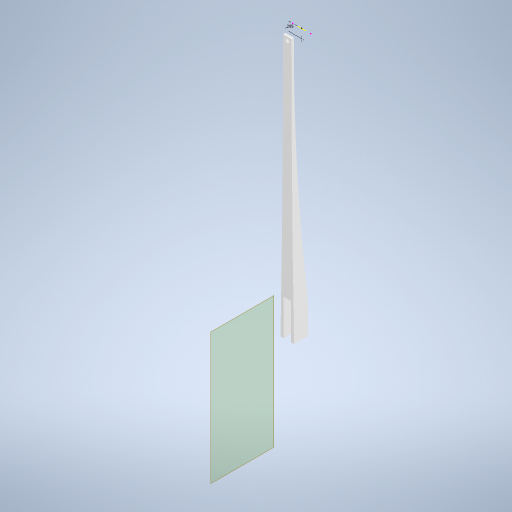
# Autodesk Inventor part: Halterung
Saved by Autodesk Inventor 2023 (Build 270158000, 158)
## iProperties
Created: 2023-02-18
Part Number: Halterung
Material: ABS Plastic
Document SubType Name: Modeling
Designer: phill
Density: 1.06 g/cm^3
Appearance: Smooth - White
Author: phill
Autodesk Inventor part; units mm, degrees
ref_plane "YZ Plane" through (0, 0, 0) normal (1, 0, 0) x (0, 1, 0)
ref_plane "XZ Plane" through (0, 0, 0) normal (0, 1, 0) x (-1, 0, 0)
sketch "Sketch2" plane through (0, 0, 0) normal (0, 0, 1) x (1, 0, 0)
  line L0 (0, 0) -> (0, -100) projected
  line L1 (0, 0) -> (6, 0) projected
  line L2 (6, -100) -> (6, 0) projected
  line L3 (0, -100) -> (6, -100) projected
  line L4 (10.5, -30) -> (-4.5, -30)
  line L5 (-4.5, -30) -> (-4.5, 190)
  line L6 (-4.5, 190) -> (10.5, 190)
  line L7 (10.5, 190) -> (10.5, -30)
  line L8 (6.5, 0.5) -> (-0.5, 0.5)
  line L9 (-0.5, 0.5) -> (-0.5, -100.5)
  line L10 (-0.5, -100.5) -> (6.5, -100.5)
  line L11 (6.5, -100.5) -> (6.5, 0.5)
  line L12 (6.5, 0.5) -> (-0.5, 0.5)
  line L13 (-0.5, 0.5) -> (-0.5, 190)
  line L14 (-0.5, 190) -> (6.5, 190)
  line L15 (6.5, 190) -> (6.5, 0.5)
  line L16 (0, -100) -> (0, 0) projected
  line L17 (0, 0) -> (6, 0) projected
  line L18 (6, 0) -> (6, -100) projected
  line L19 (-0.5, 175) -> (6.5, 175)
  line L20 (-4.5, 175) -> (-0.5, 175)
  line L21 (6.5, 175) -> (10.5, 175)
  circle A0 centre (3, -90) radius 1.5 projected
  arc A1 (-2.6174, -30) -> (-0.5, 190) centre (-11430.5, 190) ccw
  arc A2 (6.5, 190) -> (8.6174, -30) centre (11436.5, 190) ccw
  point P0 (3, -30)
  point P1 (3, 0)
  point P2 (3, 182.5)
  point P3 (3, 0)
  point P4 (3, 190)
  point P5 (3, 190)
  dimension "d0" = 30
  dimension "d1" = 15
  dimension "d2" = 220
  dimension "d3" = 0.5
  dimension "d8" = 7.5
  dimension "d10" = 22860
  dimension "d11" = 22860
  constraints: 30 end point, 5 horizontal, 5 midpoint, 4 parallel, 4 point on circle, 3 point on line, 2 centre point, 2 horizontal alignment, 2 perpendicular, 2 tangent, 2 vertical alignment, 1 coincident, 7 other
  measures "d0" distance between parallel lines of L1 L4
  measures "d1" distance between parallel lines of L5 L7
  measures "d2" distance between parallel lines of L6 L4
  measures "d3" distance between parallel lines of L11 L2
  measures "d8" distance from line of L6 point (3, 182.5)
  measures "d10" diameter of A1
  measures "d11" diameter of A2
extrude "Extrusion1" add sketch "Sketch2" against normal blind 4 contours L1 L2 L4 L0 | L0 L4 L9 L8 L11 L2 L1 | L4 A1 L20 L13 L9 | L11 L15 L21 A2 L4 | L13 L19 L15 L8 | A1 L13 L20 | L13 L6 L15 L19 | L21 L15 A2
sketch "Sketch3" plane through (0, 0, 0) normal (0, 0, 1) x (1, 0, 0)
  line L0 (10.5, -30) -> (10.5, 190) projected
  line L1 (6.5, 190) -> (6.5, 0.5) projected
  line L2 (6.5, -100.5) -> (6.5, 0.5) projected
  line L3 (-0.5, 0.5) -> (-0.5, -100.5) projected
  line L4 (-0.5, 0.5) -> (-0.5, 190) projected
  line L5 (6.5, 0.5) -> (-0.5, 0.5) projected
  line L6 (-4.5, -30) -> (10.5, -30) projected
  line L7 (-2.6174, -30) -> (8.6174, -30) projected
  line L8 (6.5, 190) -> (-0.5, 190) projected
  arc A0 (6.5, 190) -> (8.6174, -30) centre (11436.5, 190) ccw projected
  arc A1 (-2.6174, -30) -> (-0.5, 190) centre (-11430.5, 190) ccw projected
  point P0 (0, 0)
  point P1 (-0.5, -30)
  point P2 (6.5, -30)
  point P3 (-0.5, 190)
  point P4 (6.5, 190)
extrude "Extrusion2" add sketch "Sketch3" along normal blind 8
sketch "Sketch4" plane through (0, 0, -4) normal (0, 0, -1) x (-1, 0, 0)
  line L0 (0.5, 190) -> (-6.5, 190) projected
  point P0 (0, 0)
  point P1 (-3, 182.507)
  point P2 (4.5, 190)
  point P3 (-10.5, 190)
  point P4 (-3, 190)
  dimension "d9" = 7.493
  constraints: 1 midpoint, 1 vertical alignment
  measures "d9" distance from line of L0 point (-3, 182.507)
sketch "Sketch5" plane through (0, 0, -4) normal (0, 0, -1) x (-1, 0, 0)
  line L0 (-8.6174, -30) -> (2.6174, -30) projected
  line L1 (0.5, 190) -> (-6.5, 190) projected
  point P0 (0, 0)
  point P1 (-3, 187)
  point P2 (-3, -30)
  point P3 (-3, 190)
  dimension "d12" = 3
  constraints: 2 midpoint, 1 vertical alignment
  measures "d12" distance of point (-3, 190) point (-3, 187)
hole "Hole1" at (3, 187, -4) direction (0, 0, 1) diameter 3 end through all
ref_plane "Work Plane1" through (0, -50, 42.7167) normal (-1, 0, 0) x (0, 1, 0)
sketch "Sketch6" plane through (0, -50, 42.7167) normal (-1, 0, 0) x (0, 1, 0)
  arc A0 (20, 49.8247) -> (240, 36.7224) centre (235.5, 1814.7167) ccw
  line L0 (235.5, 46.7167) -> (238.5, 46.7167) projected
  line L1 (20, 46.7167) -> (240, 46.7167) projected
  line L2 (240, 46.7167) -> (20, 46.7167) projected
  line L3 (235.5, 34.7167) -> (235.5, 46.7167) projected
  line L4 (238.5, 34.7167) -> (238.5, 46.7167) projected
  line L5 (235.5, 34.7167) -> (235.5, 46.7167) projected
  line L6 (240, 46.7167) -> (240, 34.7167) projected
  line L7 (20, 46.7167) -> (240, 46.7167) projected
  line L8 (20, 34.7167) -> (20, 46.7167) projected
  line L9 (240, 34.7167) -> (20, 34.7167) projected
  point P0 (50, 42.7167)
  point P1 (47.1917, 46.7167)
  dimension "d20" = 2
  dimension "d21" = 3556
  constraints: 2 point on circle, 2 point on line, 1 centre point, 1 vertical alignment
  measures "d20" distance edge to line of A0 L9
  measures "d21" diameter of A0
extrude "Extrusion3" cut sketch "Sketch6" along normal through all both and the other way through all contours L1 L3 A0 | L3 L0 L4 A0 | L4 L1 L6 A0
sketch "Sketch7" plane through (0, 0, 8) normal (0, 0, 1) x (1, 0, 0)
  line L0 (0, 0) -> (6, 0) projected
  line L1 (0, -100) -> (0, 0) projected
  line L2 (6, 0) -> (6, -100) projected
  line L3 (-0.1, -100) -> (-0.1, 0.1)
  line L4 (-0.1, 0.1) -> (6.1, 0.1)
  line L5 (6.1, 0.1) -> (6.1, -100)
  line L6 (-2.6174, -30) -> (8.6174, -30) projected
  point P0 (0, -30)
  point P1 (6, -30)
  dimension "d24" = 0.1
  constraints: 6 end point, 2 other
  measures "d24" distance between parallel lines of L1 L3
ref_plane "Work Plane2" through (0, -100, -0.0013) normal (0, 0, -1) x (0, 1, 0)
extrude "Extrusion4" cut sketch "Sketch7" against normal up to surface (8.0013 mm away) contours L0 L2 L6 L1
equation "\"d11\" = d10"
body "Solid1"
